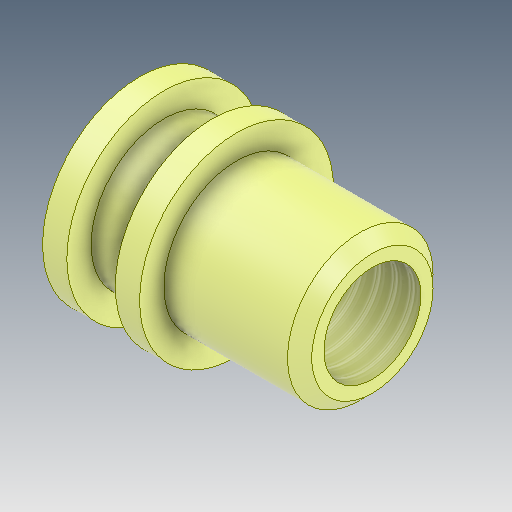
# Autodesk Inventor part: Tuerca remache m4
Saved by Autodesk Inventor 2020.3 (Build 243373000, 373)
## iProperties
Created: 2020-06-28
Part Number: Tuerca remache m4
Material: Aluminum 7175 T73 0 Hot Formed
Document SubType Name: Modeling
Designer: Pipi
Density: 2.8 g/cm^3
Appearance: Satinado - Limón gasa
Author: Pipi
Autodesk Inventor part; units mm, degrees
ref_plane "YZ Plane" through (0, 0, 0) normal (1, 0, 0) x (0, 1, 0)
ref_plane "XZ Plane" through (0, 0, 0) normal (0, 1, 0) x (-1, 0, 0)
ref_plane "XY Plane" through (0, 0, 0) normal (0, 0, 1) x (1, 0, 0)
sketch "Boceto2" plane through (0, 0, 0) normal (0, 1, 0) x (-1, 0, 0)
  line L0 (99.3538, -66.4173) -> (-152.1277, -66.4173)
  line L1 (-90.5006, -68.4173) -> (-90.5006, -69.4173)
  line L2 (-89.5006, -69.4173) -> (-89.5006, -68.4173)
  line L3 (-92.5006, -68.4173) -> (-92.5006, -69.4173)
  line L4 (-99.1006, -68.4173) -> (-99.1006, -69.4173)
  line L5 (-99.1006, -69.4173) -> (-93.5006, -69.4173)
  line L6 (-93.5006, -70.4173) -> (-92.5006, -70.4173)
  line L7 (-92.5006, -70.4173) -> (-92.5006, -69.4173)
  line L8 (-90.5006, -69.4173) -> (-90.5006, -70.4173)
  line L9 (-90.5006, -70.4173) -> (-89.5006, -70.4173)
  line L10 (-89.5006, -70.4173) -> (-89.5006, -69.4173)
  line L11 (-93.5006, -68.4173) -> (-93.5006, -70.4173)
  line L12 (-92.5006, -69.4173) -> (-90.5006, -69.4173)
  line L13 (-99.1006, -68.4173) -> (-89.5006, -68.4173)
  point P0 (0, 0)
  dimension "d17" = 1
  constraints: 28 end point, 5 perpendicular, 5 point on line, 2 horizontal, 2 parallel, 1 vertical
  measures "d17" distance of L1.end L2.start
revolve "Revolución1" add sketch "Boceto2" angle 360 about axis through (-99.3538, 0, -66.4173) along (1, 0, 0)
chamfer "Chaflán2" distance 0.5 angle 45 1 edges at (99.1006, 0, -63.4173)
sketch "Boceto3" plane through (89.5006, 0, -66.4173) normal (-1, 0, 0) x (0, 0, 1)
  circle A0 centre (0, 0) radius 2.625
  point P0 (66.4173, 0)
  dimension "d28" = 5.25
  constraints: 1 centre point
  measures "d28" diameter of A0
extrude "Extrusión3" cut sketch "Boceto3" against normal blind 2.5
thread "Rosca3" size "M4x0.7" class "6H" standard "ISO Metric profile" length 7
